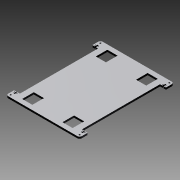
# Autodesk Inventor part: BED PLATE BOTTOM
Saved by Autodesk Inventor 2013 (Build 170138000, 138)
## iProperties
Created: 2014-06-19
Part Number: BED PLATE BOTTOM
Material: Generic
Document SubType Name: Modeling
Designer: employee
Density: 1 g/cm^3
Author: employee
Autodesk Inventor part; units mm, degrees
ref_plane "YZ Plane" through (0, 0, 0) normal (1, 0, 0) x (0, 1, 0)
ref_plane "XZ Plane" through (0, 0, 0) normal (0, 1, 0) x (-1, 0, 0)
ref_plane "XY Plane" through (0, 0, 0) normal (0, 0, 1) x (1, 0, 0)
sketch "Sketch1" plane through (0, 0, 0) normal (0, 0, 1) x (1, 0, 0)
  line L0 (0, 0) -> (-107, 0)
  line L1 (-107, 0) -> (-107, 135)
  line L2 (-107, 135) -> (-115, 135)
  line L3 (-115, 135) -> (-115, 145)
  line L4 (-115, 145) -> (-119, 145)
  line L5 (-119, 145) -> (-119, 135)
  line L6 (-119, 135) -> (-127, 135)
  line L7 (-127, 135) -> (-127, 155)
  arc A0 (-119, 163) -> (-127, 155) centre (-119, 155) ccw
  line L8 (-119, 163) -> (0, 163)
  line L9 (0, 163) -> (0, 0)
  circle A1 centre (-119, 155) radius 2.5
  line L10 (-122.5, 142) -> (-121, 142)
  line L11 (-121, 142) -> (-121, 138)
  line L12 (-121, 138) -> (-122.5, 138)
  line L13 (-122.5, 138) -> (-122.5, 142)
  line L14 (-113, 142) -> (-111.5, 142)
  line L15 (-111.5, 142) -> (-111.5, 138)
  line L16 (-111.5, 138) -> (-113, 138)
  line L17 (-113, 138) -> (-113, 142)
  line L18 (-87, 147) -> (-52, 147)
  line L19 (-52, 147) -> (-52, 107)
  line L20 (-52, 107) -> (-87, 107)
  line L21 (-87, 107) -> (-87, 147)
  point P0 (-117, 145)
  point P1 (-121, 140)
  point P2 (-119, 140)
  point P3 (-113, 140)
  point P4 (-115, 140)
  point P5 (-52, 127)
  dimension "d1" = 145
  dimension "d3" = 4
  dimension "d4" = 10
  dimension "d5" = 10
  dimension "d6" = 10
  dimension "d7" = 127
  dimension "d8" = 8
  dimension "d9" = 10
  dimension "d10" = 5
  dimension "d14" = 4
  dimension "d15" = 8
  dimension "d16" = 1.5
  dimension "d17" = 4
  dimension "d18" = 40
  dimension "d19" = 35
  dimension "d20" = 127
  dimension "d21" = 20
  constraints: 44 end point, 14 parallel, 6 midpoint, 4 horizontal, 4 perpendicular, 3 horizontal alignment, 2 centre point, 2 equal length, 2 point on circle, 2 tangent, 1 coincident
  measures "d1" distance from line of L4.end L0
  measures "d3" distance between parallel lines of L3 L5
  measures "d4" distance of L2.end L3.end
  measures "d5" distance from line of L1 point (-117, 145)
  measures "d6" distance from line of L7 point (-117, 145)
  measures "d7" distance between parallel lines of L7 L9
  measures "d8" radius of A0
  measures "d9" vertical distance of point (-117, 145) A0.centre
  measures "d10" diameter of A1
  measures "d14" distance from line of point (-117, 145) L11
  measures "d15" distance between parallel lines of L17 L11
  measures "d16" distance of L15.end L16.end
  measures "d17" distance of L14.end L15.end
  measures "d18" distance of L18.end L19.end
  measures "d19" distance of L19.end L20.end
  measures "d20" distance from line of L0 point (-52, 127)
  measures "d21" distance between parallel lines of L21 L1
extrude "Extrusion1" add sketch "Sketch1" along normal blind 6.477
fillet "Fillet1" radius 2 2 edges at (-107, 135, 3.2385) (-127, 135, 3.2385)
mirror "Mirror1" about plane through (-107, 0, 0) normal (0, -1, 0) of "Extrusion1", "Fillet1"
mirror "Mirror2" about plane through (0, 0, 0) normal (1, 0, 0) of "Extrusion1", "Mirror1", "Fillet1"
sketch "Sketch2" plane through (0, 0, 6.477) normal (0, 0, 1) x (1, 0, 0)
  arc A0 (5, 118) -> (10, 113) centre (10, 118) ccw projected
  line L0 (10, 113) -> (113, 113) projected
  line L1 (113, 113) -> (113, -113) projected
  line L2 (113, -113) -> (-113, -113) projected
  line L3 (-113, -113) -> (-113, 113) projected
  line L4 (-113, 113) -> (-10, 113) projected
  arc A1 (-10, 113) -> (-5, 118) centre (-10, 118) ccw projected
  line L5 (-5, 118) -> (-5, 142) projected
  arc A2 (5, 142) -> (-5, 142) centre (0, 142) ccw projected
  line L6 (5, 142) -> (5, 118) projected
  line L7 (-52, 147) -> (-52, 127) projected
  line L8 (-52, 127) -> (-87, 127) projected
  line L9 (-87, 127) -> (-87, 147) projected
  line L10 (-87, 147) -> (-52, 147) projected
  line L11 (-52, -147) -> (-87, -147) projected
  line L12 (-87, -147) -> (-87, -127) projected
  line L13 (-87, -127) -> (-52, -127) projected
  line L14 (-52, -127) -> (-52, -147) projected
  line L15 (52, 147) -> (87, 147) projected
  line L16 (87, 147) -> (87, 127) projected
  line L17 (87, 127) -> (52, 127) projected
  line L18 (52, 127) -> (52, 147) projected
  line L19 (52, -147) -> (52, -127) projected
  line L20 (52, -127) -> (87, -127) projected
  line L21 (87, -127) -> (87, -147) projected
  line L22 (87, -147) -> (52, -147) projected
  circle A3 centre (-119, 155) radius 2.5 projected
  circle A4 centre (-119, -155) radius 2.5 projected
  circle A5 centre (119, 155) radius 2.5 projected
  circle A6 centre (119, -155) radius 2.5 projected
  line L23 (-121, 138) -> (-122.5, 138) projected
  line L24 (-122.5, 138) -> (-122.5, 142) projected
  line L25 (-122.5, 142) -> (-121, 142) projected
  line L26 (-121, 142) -> (-121, 138) projected
  line L27 (-111.5, 138) -> (-113, 138) projected
  line L28 (-113, 138) -> (-113, 142) projected
  line L29 (-113, 142) -> (-111.5, 142) projected
  line L30 (-111.5, 142) -> (-111.5, 138) projected
  line L31 (-111.5, -142) -> (-113, -142) projected
  line L32 (-113, -142) -> (-113, -138) projected
  line L33 (-113, -138) -> (-111.5, -138) projected
  line L34 (-111.5, -138) -> (-111.5, -142) projected
  line L35 (-121, -142) -> (-122.5, -142) projected
  line L36 (-122.5, -142) -> (-122.5, -138) projected
  line L37 (-122.5, -138) -> (-121, -138) projected
  line L38 (-121, -138) -> (-121, -142) projected
  line L39 (111.5, 142) -> (113, 142) projected
  line L40 (113, 142) -> (113, 138) projected
  line L41 (113, 138) -> (111.5, 138) projected
  line L42 (111.5, 138) -> (111.5, 142) projected
  line L43 (121, 142) -> (122.5, 142) projected
  line L44 (122.5, 142) -> (122.5, 138) projected
  line L45 (122.5, 138) -> (121, 138) projected
  line L46 (121, 138) -> (121, 142) projected
  line L47 (111.5, -138) -> (113, -138) projected
  line L48 (113, -138) -> (113, -142) projected
  line L49 (113, -142) -> (111.5, -142) projected
  line L50 (111.5, -142) -> (111.5, -138) projected
  line L51 (121, -138) -> (122.5, -138) projected
  line L52 (122.5, -138) -> (122.5, -142) projected
  line L53 (122.5, -142) -> (121, -142) projected
  line L54 (121, -142) -> (121, -138) projected
  line L55 (-127, 155) -> (-127, -155) projected
  arc A7 (-127, -155) -> (-119, -163) centre (-119, -155) ccw projected
  line L56 (-119, -163) -> (119, -163) projected
  arc A8 (119, -163) -> (127, -155) centre (119, -155) ccw projected
  line L57 (127, -155) -> (127, 155) projected
  arc A9 (127, 155) -> (119, 163) centre (119, 155) ccw projected
  line L58 (119, 163) -> (-119, 163) projected
  arc A10 (-119, 163) -> (-127, 155) centre (-119, 155) ccw projected
  line L59 (-12.5, 113) -> (-12.5, 100.5)
  arc A11 (-12.5, 100.5) -> (12.5, 100.5) centre (0, 100.5) ccw
  line L60 (12.5, 100.5) -> (12.5, 113)
  point P0 (0, 0)
  dimension "d22" = 12.5
  dimension "d24" = 12.5
  constraints: 4 end point, 2 perpendicular, 2 point on circle, 2 point on line, 2 tangent, 1 centre point, 1 vertical alignment
  measures "d22" distance of L60.start L60.end
  measures "d24" radius of A11
extrude "Extrusion2" cut sketch "Sketch2" against normal through all contours A0 L0 L60 A11 L59 L4 A1 L5 A2 L6
body "Solid1"
